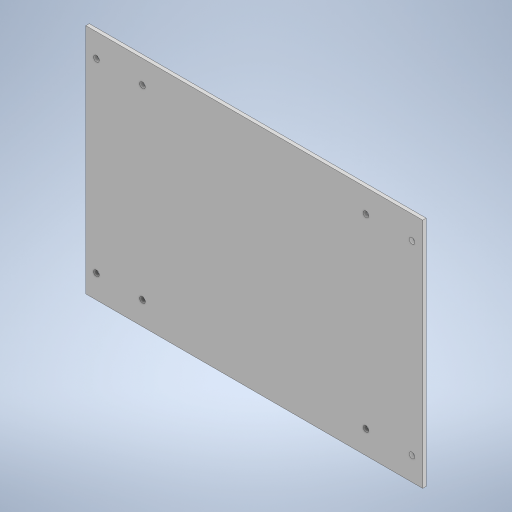
# Autodesk Inventor part: base
Saved by Autodesk Inventor 2024 (Build 280153000, 153)
## iProperties
Created: 2024-03-16
Part Number: base
Material: Generic
Document SubType Name: Modeling
Designer: op04o
Density: 1 g/cm^3
Appearance: Default
Author: op04o
Autodesk Inventor part; units mm, degrees
ref_plane "YZ Plane" through (0, 0, 0) normal (1, 0, 0) x (0, 1, 0)
ref_plane "XZ Plane" through (0, 0, 0) normal (0, 1, 0) x (-1, 0, 0)
ref_plane "XY Plane" through (0, 0, 0) normal (0, 0, 1) x (1, 0, 0)
sketch "Sketch1" plane through (0, 0, 0) normal (0, 0, 1) x (1, 0, 0)
  line L0 (0, 0) -> (290, 0)
  line L1 (290, 0) -> (290, 200)
  line L2 (290, 200) -> (0, 200)
  line L3 (0, 200) -> (0, 0)
  line L4 (9.2, 180) -> (48.8, 180)
  circle A0 centre (9.2, 180) radius 2.5
  circle A1 centre (48.8, 180) radius 2.5
  line L5 (0, 100) -> (290, 100)
  line L6 (9.2, 20) -> (48.8, 20)
  circle A2 centre (9.2, 20) radius 2.5
  circle A3 centre (48.8, 20) radius 2.5
  line L7 (241.2, 180) -> (280.8, 180)
  circle A4 centre (241.2, 180) radius 2.5
  circle A5 centre (280.8, 180) radius 2.5
  line L8 (241.2, 20) -> (280.8, 20)
  circle A6 centre (241.2, 20) radius 2.5
  circle A7 centre (280.8, 20) radius 2.5
  dimension "d0" = 290
  dimension "d1" = 200
  dimension "d2" = 39.6
  dimension "d4" = 9.2
  dimension "d5" = 20
  dimension "d6" = 5
  dimension "d8" = 5
  dimension "d13" = 39.6
  dimension "d14" = 5
  dimension "d15" = 5
  dimension "d16" = 9.2
  dimension "d17" = 20
  constraints: 18 end point, 8 centre point, 8 coincident, 8 symmetric about line, 3 horizontal, 2 midpoint, 2 parallel, 1 perpendicular, 4 other
  measures "d0" distance of L2.end L1.end
  measures "d1" distance of L1.end L0.end
  measures "d2" distance of L4.start L4.end
  measures "d4" distance from line of L3 L4.start
  measures "d5" distance from line of L4.end L2
  measures "d6" diameter of A0
  measures "d8" diameter of A1
  measures "d13" distance of L7.start L7.end
  measures "d14" diameter of A4
  measures "d15" diameter of A5
  measures "d16" distance from line of L1 L7.end
  measures "d17" distance between parallel lines of L2 L7
extrude "Extrusion1" add sketch "Sketch1" along normal blind 3
body "Solid1"
